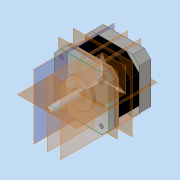
# Autodesk Inventor part: NEMA-7-17HD34008-22B
Saved by Autodesk Inventor 2016 SP1 (Build 200210100, 210)
## iProperties
Created: 2015-11-14
Part Number: NEMA-7-17HD34008-22B
Material: Aluminum 6061
Document SubType Name: Modeling
Designer: Mohamed A.
Density: 2.7 g/cm^3
Appearance: Aluminum - Dark
Mass: 149.241 g
Surface Area: 158.856 cm^2
Volume: 55.2745 cm^3
Author: Mohamed A.
Autodesk Inventor part; units mm, degrees
ref_plane "YZ Plane" through (0, 0, 0) normal (1, 0, 0) x (0, 1, 0)
ref_plane "XY Plane" through (0, 0, 0) normal (0, 0, 1) x (1, 0, 0)
sketch "Sketch1" plane through (0, 0, 0) normal (0, 0, 1) x (1, 0, 0)
  line L0 (21, 21) -> (21, -21)
  line L1 (21, -21) -> (-21, -21)
  line L2 (-21, -21) -> (-21, 21)
  line L3 (-21, 21) -> (21, 21)
  point P0 (0, 0)
  point P1 (0, 0)
  dimension "d0" = 42
  constraints: 8 end point, 1 coincident, 1 horizontal, 9 other
  measures "d0" distance of L0.start L0.end
extrude "Extrusion1" add sketch "Sketch1" along normal blind 8
chamfer "Chamfer1" distance 5 angle 45 4 edges at (21, 21, 4) (-21, 21, 4) (-21, -21, 4) (21, -21, 4)
sketch "Sketch2" plane through (0, 0, 8) normal (0, 0, 1) x (1, 0, 0)
  circle A0 centre (0, 0) radius 11
  dimension "d6" = 22
  constraints: 1 centre point, 1 coincident
  measures "d6" diameter of A0
extrude "Extrusion2" add sketch "Sketch2" along normal blind 2
sketch "Sketch3" plane through (0, 0, 10) normal (0, 0, 1) x (1, 0, 0)
  circle A0 centre (0, 0) radius 5
  dimension "d9" = 10
  constraints: 1 centre point, 1 coincident
  measures "d9" diameter of A0
extrude "Extrusion3" cut sketch "Sketch3" against normal blind 3
sketch "Sketch4" plane through (0, 0, 7) normal (0, 0, 1) x (1, 0, 0)
  circle A0 centre (0, 0) radius 2.5
  dimension "d12" = 5
  constraints: 1 centre point, 1 coincident
  measures "d12" diameter of A0
extrude "Extrusion4" add sketch "Sketch4" along normal blind 25
ref_plane "Work Plane2" through (0, 0, 3) normal (0, 0, 1) x (1, 0, 0)
sketch "Sketch6" plane through (0, 0, 8) normal (0, 0, 1) x (1, 0, 0)
  line L0 (16, 21) -> (-16, 21) projected
  line L1 (21, -16) -> (21, 16) projected
  line L2 (-16, -21) -> (16, -21) projected
  line L3 (-21, 16) -> (-21, -16) projected
  point P0 (0, 0)
  point P1 (15.5, 15.5)
  point P2 (-15.5, 15.5)
  point P3 (-15.5, -15.5)
  point P4 (15.5, -15.5)
  dimension "d59" = 31
  dimension "d60" = 5.5
  dimension "d61" = 5.5
  dimension "d62" = 5.5
  dimension "d63" = 5.5
  dimension "d64" = 5.5
  dimension "d65" = 5.5
  measures "d59" distance of point (-15.5, 15.5) point (15.5, 15.5)
  measures "d60" distance from line of L0 point (15.5, 15.5)
  measures "d61" distance from line of L1 point (15.5, 15.5)
  measures "d62" distance from line of L1 point (15.5, -15.5)
  measures "d63" distance from line of L2 point (15.5, -15.5)
  measures "d64" distance from line of L2 point (-15.5, -15.5)
  measures "d65" distance from line of L3 point (-15.5, -15.5)
hole "Hole1" [suppressed]
sketch "Sketch7" plane through (0, 0, 0) normal (0, 0, -1) x (-1, 0, 0)
  line L0 (-21, -21) -> (21, -21)
  line L1 (21, -21) -> (21, 21)
  line L2 (21, 21) -> (-21, 21)
  line L3 (-21, 21) -> (-21, -21)
  line L4 (-21, -21) -> (21, 21) construction
  line L5 (21, -21) -> (-21, 21) construction
  point P0 (0, 0)
  dimension "d30" = 42
  dimension "d31" = 42
  constraints: 12 end point, 2 midpoint, 2 parallel, 1 horizontal, 1 perpendicular
  measures "d30" distance of L2.end L1.end
  measures "d31" distance of L1.end L0.end
extrude "Extrusion5" add sketch "Sketch7" along normal blind 16 separate body
chamfer "Chamfer3" distance 10 angle 45 4 edges at (-21, 21, -8) (-21, -21, -8) (21, 21, -8) (21, -21, -8)
sketch "Sketch8" plane through (0, 0, -16) normal (0, 0, -1) x (-1, 0, 0)
  line L0 (-21, -21) -> (21, -21)
  line L1 (21, -21) -> (21, 21)
  line L2 (21, 21) -> (-21, 21)
  line L3 (-21, 21) -> (-21, -21)
  line L4 (-21, -21) -> (21, 21) construction
  line L5 (21, -21) -> (-21, 21) construction
  point P0 (0, 0)
  dimension "d37" = 42
  dimension "d38" = 42
  constraints: 12 end point, 2 midpoint, 2 parallel, 1 horizontal, 1 perpendicular
  measures "d37" distance of L2.end L1.end
  measures "d38" distance of L1.end L0.end
extrude "Extrusion6" add sketch "Sketch8" along normal blind 9 separate body
chamfer "Chamfer4" distance 5 angle 45 4 edges at (21, 21, -20.5) (21, -21, -20.5) (-21, -21, -20.5) (-21, 21, -20.5)
sketch "Sketch9" plane through (-16, -21, -16) normal (0, -1, 0) x (1, 0, 0)
  line L0 (32, -9) -> (0, -9) projected
  line L1 (0, -9) -> (0, 0) projected
  line L2 (32, -9) -> (0, -9) projected
  line L3 (32, 0) -> (32, -9) projected
  line L4 (32, 0) -> (0, 0) projected
  line L5 (32, 0) -> (0, 0) projected
  line L6 (24, -9) -> (8, -9)
  line L7 (8, -9) -> (8, 0)
  line L8 (8, 0) -> (24, 0)
  line L9 (24, 0) -> (24, -9)
  line L10 (24, -9) -> (8, 0) construction
  line L11 (8, -9) -> (24, 0) construction
  point P0 (16, 16)
  point P1 (16, -4.5)
  dimension "d44" = 16
  constraints: 12 end point, 2 midpoint, 2 parallel, 1 horizontal, 1 perpendicular, 1 point on line
  measures "d44" distance of L7.end L8.end
extrude "Extrusion7" add sketch "Sketch9" along normal blind 4 contours L0 L7 L4 L9 bodies 3
sketch "Sketch10" plane through (-16, -25, -16) normal (0, -1, 0) x (1, 0, 0)
  line L0 (8, 0) -> (8, -9) projected
  line L1 (8, -9) -> (24, -9) projected
  line L2 (24, -9) -> (24, 0) projected
  line L3 (24, 0) -> (8, 0) projected
  line L4 (8, -6) -> (24, -6)
  line L5 (24, -6) -> (24, 0)
  line L6 (24, 0) -> (8, 0)
  line L7 (8, 0) -> (8, -6)
  line L8 (8, -6) -> (24, 0) construction
  line L9 (24, -6) -> (8, 0) construction
  point P0 (16, 16)
  point P1 (16, -3)
  dimension "d47" = 3
  constraints: 12 end point, 2 midpoint, 2 parallel, 1 horizontal, 1 perpendicular
  measures "d47" distance between parallel lines of L1 L4
extrude "Extrusion8" cut sketch "Sketch10" against normal blind 4 contours L3 L2 L4 L0 bodies 3
ref_plane "Work Plane1" through (0, 0, 0) normal (0, 1, 0) x (-1, 0, 0)
ref_plane "Work Plane3" through (0, 0, -8.5) normal (0, 0, 1) x (1, 0, 0)
hole "Hole8" [suppressed]
split body "Split1" result two bodies by plane through (0, 0, 3) normal (0, 0, 1) bodies 1 first body at (3.6667, -5.3333, 3.5)
hole "Hole12" at (15.5, -15.5, 8) at (-15.5, -15.5, 8) at (-15.5, 15.5, 8) at (15.5, 15.5, 8) direction (0, 0, -1) diameter 3 depth 4.5 bodies 4
sketch "Sketch15" plane through (16, 21, 3) normal (0, 0, -1) x (-1, 0, 0)
  point P0 (0.5, -5.5)
  point P1 (31.5, -5.5)
  point P2 (31.5, -36.5)
  point P3 (0.5, -36.5)
sketch "Sketch17" plane through (16, 21, 3) normal (0, 0, -1) x (-1, 0, 0)
  point P0 (31.5, -5.5)
  point P1 (31.5, -36.5)
  point P2 (0.5, -5.5)
  point P3 (0.5, -36.5)
hole "Hole13" at (-15.5, 15.5, 3) at (-15.5, -15.5, 3) at (15.5, 15.5, 3) at (15.5, -15.5, 3) direction (0, 0, 1) diameter 5.3 depth 0.5 bodies 4
ref_plane "Work Plane4" through (0, -16, -16) normal (1, 0, 0) x (0, 0, -1)
ref_plane "Work Plane5" through (0, 0, 0) normal (0, 1, 0) x (-1, 0, 0)
ref_plane "Work Plane6" through (10.5, -16, -16) normal (1, 0, 0) x (0, 0, -1)
ref_plane "Work Plane7" through (-10.5, -16, -16) normal (-1, 0, 0) x (0, 0, 1)
equation "\"d61\" = d60"
equation "\"d62\" = d60"
equation "\"d63\" = d62"
equation "\"d64\" = d62"
equation "\"d65\" = d62"
body "Solid2"
body "Solid3"
body "Solid4"
body "Solid5"
